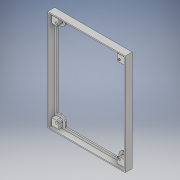
# Autodesk Inventor part: TestTapa_v1
Saved by Autodesk Inventor 2019 (Build 230136000, 136)
## iProperties
Created: 2019-05-27
Part Number: TestTapa_v1
Material: Genérico
Document SubType Name: Modeling
Designer: LuisAlonso
Density: 1 g/cm^3
Appearance: Valor por defecto
Author: LuisAlonso
Autodesk Inventor part; units mm, degrees
ref_plane "YZ Plane" through (0, 0, 0) normal (1, 0, 0) x (0, 1, 0)
ref_plane "XZ Plane" through (0, 0, 0) normal (0, 1, 0) x (-1, 0, 0)
ref_plane "XY Plane" through (0, 0, 0) normal (0, 0, 1) x (1, 0, 0)
sketch "Boceto1" plane through (0, 0, 0) normal (0, 0, 1) x (1, 0, 0)
  line L0 (-83, -108.2) -> (83, -108.2)
  line L1 (83, -108.2) -> (83, 108.2)
  line L2 (83, 108.2) -> (-83, 108.2)
  line L3 (-83, 108.2) -> (-83, -108.2)
  line L4 (-83, -108.2) -> (83, 108.2) construction
  line L5 (83, -108.2) -> (-83, 108.2) construction
  point P0 (0, 0)
  dimension "d0" = 166
  dimension "d1" = 216.4
  constraints: 12 end point, 2 midpoint, 2 parallel, 1 horizontal, 1 perpendicular
  measures "d0" distance of L2.end L1.end
  measures "d1" distance of L1.end L0.end
extrude "Extrusión1" add sketch "Boceto1" along normal blind 15
sketch "Boceto2" plane through (0, 0, 15) normal (0, 0, 1) x (1, 0, 0)
  line L0 (80.75, -105.95) -> (-80.75, -105.95)
  line L1 (-80.75, -105.95) -> (-80.75, 105.95)
  line L2 (80.75, 105.95) -> (-80.75, 105.95)
  line L3 (80.75, 105.95) -> (80.75, -105.95)
  line L4 (-83, 108.2) -> (83, 108.2)
  line L5 (83, 108.2) -> (83, -108.2)
  line L6 (83, -108.2) -> (-83, -108.2)
  line L7 (-83, -108.2) -> (-83, 108.2)
  point P0 (0, 0)
  constraints: 16 end point, 4 perpendicular, 2 parallel, 1 horizontal
extrude "Extrusión2" cut sketch "Boceto2" against normal blind 12 contours L0 L1 L2 L3
sketch "Boceto3" plane through (0, 0, 3) normal (0, 0, 1) x (1, 0, 0)
  line L0 (-67.5, -92.5) -> (67.5, -92.5)
  line L1 (67.5, -92.5) -> (67.5, 92.5)
  line L2 (67.5, 92.5) -> (-67.5, 92.5)
  line L3 (-67.5, 92.5) -> (-67.5, -92.5)
  line L4 (-67.5, 87.5) -> (-72.5, 87.5)
  line L5 (-62.5, 97.5) -> (-62.5, 92.5)
  line L6 (62.5, -97.5) -> (62.5, -92.5)
  line L7 (67.5, -87.5) -> (72.5, -87.5)
  line L8 (-72.5, -87.5) -> (-67.5, -87.5)
  line L9 (-62.5, -92.5) -> (-62.5, -97.5)
  line L10 (-72.5, 87.5) -> (-77.5, 87.5)
  line L11 (-77.5, 87.5) -> (-77.5, 102.5)
  line L12 (-77.5, 102.5) -> (-62.5, 102.5)
  line L13 (-62.5, 102.5) -> (-62.5, 97.5)
  line L14 (77.5, 87.5) -> (77.5, 102.5)
  line L15 (77.5, 102.5) -> (62.5, 102.5)
  line L16 (67.5, -87.5) -> (77.5, -87.5)
  line L17 (62.5, -92.5) -> (62.5, -102.5)
  line L18 (62.5, -102.5) -> (77.5, -102.5)
  line L19 (77.5, -102.5) -> (77.5, -87.5)
  line L20 (-67.5, -87.5) -> (-77.5, -87.5)
  line L21 (-77.5, -87.5) -> (-77.5, -102.5)
  line L22 (-77.5, -102.5) -> (-62.5, -102.5)
  line L23 (-62.5, -102.5) -> (-62.5, -97.5)
  line L24 (67.5, 87.5) -> (77.5, 87.5)
  line L25 (62.5, 102.5) -> (62.5, 92.5)
  arc A0 (-62.5, -92.5) -> (-67.5, -87.5) centre (-67.5, -92.5) ccw
  arc A1 (-67.5, 87.5) -> (-62.5, 92.5) centre (-67.5, 92.5) ccw
  arc A2 (62.5, 92.5) -> (67.5, 87.5) centre (67.5, 92.5) ccw
  arc A3 (67.5, -87.5) -> (62.5, -92.5) centre (67.5, -92.5) ccw
  point P0 (0, 0)
  dimension "d12" = 135
  dimension "d13" = 185
  dimension "d56" = 5
  dimension "d57" = 15
  dimension "d58" = 15
  constraints: 52 end point, 10 perpendicular, 8 point on circle, 6 point on line, 4 centre point, 4 coincident, 4 horizontal, 3 vertical, 2 midpoint, 1 collinear
  measures "d12" distance of L0.start L0.end
  measures "d13" distance of L0.end L1.end
  measures "d56" distance of L4.end L10.end
  measures "d57" distance of L10.end L11.end
  measures "d58" distance of L11.end L12.end
extrude "Extrusión3" add sketch "Boceto3" along normal blind 9 contours L3 A0 L0 | L0 L9 L23 L22 L21 L20 L8 L3 | A3 L1 L0 | L0 L1 L7 L16 L19 L18 L17 L6 | L4 L10 L11 L12 L13 L5 L2 L3 | L3 L2 A1 | A2 L2 L1 | L1 L2 L25 L15 L14 L24
sketch "Boceto4" plane through (0, 0, 0) normal (0, 0, -1) x (-1, 0, 0)
  line L0 (80.75, -105.95) -> (80.75, 105.95) projected
  line L1 (-80.75, -105.95) -> (80.75, -105.95) projected
  line L2 (-80.75, 105.95) -> (-80.75, -105.95) projected
  line L3 (80.75, 105.95) -> (-80.75, 105.95) projected
  line L4 (-67.5, -92.5) -> (-67.5, 92.5) projected
  line L5 (67.5, 92.5) -> (67.5, -92.5) projected
  line L6 (-67.5, 92.5) -> (67.5, 92.5) projected
  line L7 (67.5, -92.5) -> (-67.5, -92.5) projected
  circle A0 centre (-67.5, 92.5) radius 4.75
  circle A1 centre (67.5, 92.5) radius 4.75
  circle A2 centre (67.5, -92.5) radius 4.75
  circle A3 centre (-67.5, -92.5) radius 4.75
  point P0 (0, 0)
  dimension "d24" = 9.5
  dimension "d25" = 9.5
  dimension "d26" = 9.5
  dimension "d27" = 9.5
  constraints: 4 centre point, 4 coincident
  measures "d24" diameter of A0
  measures "d25" diameter of A1
  measures "d26" diameter of A2
  measures "d27" diameter of A3
extrude "Extrusión4" cut sketch "Boceto4" against normal blind 4.5 contours L7 A3 L4 | L4 A3 L7 | A0 L6 L4 | L4 L6 A0 | A2 L5 L7 | L7 L5 A2 | A1 L5 L6 | L6 L5 A1
sketch "Boceto7" plane through (-67.5, 92.5, 4.5) normal (0, 0, -1) x (-1, 0, 0)
  arc A0 (-0.8744, -2.2886) -> (-2.2886, -0.8744) centre (0, 0) ccw
  line L0 (0, 0) -> (4.75, 0) construction
  line L1 (-2.2886, -0.8744) -> (-3.9906, -2.5764)
  line L2 (-0.8744, -2.2886) -> (-2.5764, -3.9906)
  arc A1 (-3.9906, -2.5764) -> (-2.5764, -3.9906) centre (0, 0) ccw
  arc A2 (-132.7114, -0.8744) -> (-134.1256, -2.2886) centre (-135, 0) ccw
  line L3 (-134.1256, -2.2886) -> (-132.4236, -3.9906)
  line L4 (-132.7114, -0.8744) -> (-131.0094, -2.5764)
  arc A3 (-132.4236, -3.9906) -> (-131.0094, -2.5764) centre (-135, 0) ccw
  arc A4 (-134.1256, -182.7114) -> (-132.7114, -184.1256) centre (-135, -185) ccw
  line L5 (-132.7114, -184.1256) -> (-131.0094, -182.4236)
  line L6 (-134.1256, -182.7114) -> (-132.4236, -181.0094)
  arc A5 (-131.0094, -182.4236) -> (-132.4236, -181.0094) centre (-135, -185) ccw
  arc A6 (-2.2886, -184.1256) -> (-0.8744, -182.7114) centre (0, -185) ccw
  line L7 (-0.8744, -182.7114) -> (-2.5764, -181.0094)
  line L8 (-2.2886, -184.1256) -> (-3.9906, -182.4236)
  arc A7 (-2.5764, -181.0094) -> (-3.9906, -182.4236) centre (0, -185) ccw
  point P0 (-67.5, -92.5)
  constraints: 18 end point, 16 point on circle, 8 centre point, 1 horizontal
extrude "Extrusión7" cut sketch "Boceto7" against normal blind 10
sketch "Boceto8" plane through (0, 0, 3) normal (0, 0, 1) x (1, 0, 0)
  line L0 (80.75, -105.95) -> (-80.75, -105.95) projected
  line L1 (-62.5, -105.95) -> (-57.5, -105.95)
  line L2 (-57.5, -100.95) -> (57.5161, -100.95)
  line L3 (67.5, -87.5) -> (77.5, -87.5) projected
  line L4 (57.5161, -92.5) -> (57.5161, -100.95)
  line L5 (-57.5, -100.95) -> (-57.5, -92.5)
  line L6 (-67.5, -82.5) -> (-75.75, -82.5)
  line L7 (-77.5, 87.5) -> (-67.5, 87.5) projected
  line L8 (-62.5, 92.5) -> (-62.5, 102.5) projected
  line L9 (-80.75, 105.95) -> (80.75, 105.95) projected
  line L10 (-75.75, 82.5) -> (-67.5, 82.5)
  line L11 (-57.5, 92.5) -> (-57.5, 100.95)
  line L12 (-75.75, -82.5) -> (-75.75, 82.5)
  line L13 (-57.5, 100.95) -> (57.5161, 100.95)
  line L14 (57.5161, 100.95) -> (57.5161, 91.9319)
  line L15 (67.5, 82.5) -> (75.75, 82.5)
  line L16 (75.75, 82.5) -> (75.75, -82.5161)
  arc A0 (65.2114, -91.6256) -> (66.6256, -90.2114) centre (67.5, -92.5) ccw projected
  line L17 (67.5, -82.5161) -> (75.75, -82.5161)
  arc A1 (-66.6256, -90.2114) -> (-65.2114, -91.6256) centre (-67.5, -92.5) ccw projected
  arc A2 (-57.5, -92.5) -> (-67.5, -82.5) centre (-67.5, -92.5) ccw
  arc A3 (-65.2114, 91.6256) -> (-66.6256, 90.2114) centre (-67.5, 92.5) ccw projected
  arc A4 (-67.5, 82.5) -> (-57.5, 92.5) centre (-67.5, 92.5) ccw
  arc A5 (67.5, -82.5161) -> (57.5161, -92.5) centre (67.5, -92.5) ccw
  arc A6 (66.6256, 90.2114) -> (65.2114, 91.6256) centre (67.5, 92.5) ccw projected
  arc A7 (57.5, 92.5) -> (67.5, 82.5) centre (67.5, 92.5) ccw
  point P0 (0, 0)
  constraints: 26 end point, 9 point on circle, 4 centre point, 4 coincident, 4 horizontal, 4 perpendicular, 2 point on line, 2 vertical
extrude "Extrusión8" cut sketch "Boceto8" against normal blind 10
